Autodesk Fusion 360 part; units mm, degrees
note: some values were not read from the file. Set by a fixed rule: which sketch regions a step uses.
(part 2 of 2)
sketch "Sketch33" plane through (-2.5, 0, 0) normal (-1, 0, 0) x (0, 0, 1)
  circle A0 centre (22.5, 52.5) radius 3.5
  line L0 (35.5, 59.8175) -> (35.5, 45.1825)
  line L1 (35.5, 45.1825) -> (26.719, 52.5)
  line L2 (26.719, 52.5) -> (35.5, 59.8175)
  line L3 (9.5, 59.8175) -> (18.281, 52.5)
  line L4 (18.281, 52.5) -> (9.5, 45.1825)
  line L5 (9.5, 45.1825) -> (9.5, 59.8175)
  line L6 (29.8175, 39.5) -> (15.1825, 39.5)
  line L7 (15.1825, 39.5) -> (22.5, 48.281)
  line L8 (22.5, 48.281) -> (29.8175, 39.5)
  line L9 (22.5, 56.719) -> (15.1825, 65.5)
  line L10 (15.1825, 65.5) -> (29.8175, 65.5)
  line L11 (29.8175, 65.5) -> (22.5, 56.719)
  circle A1 centre (38.5, 65) radius 0.9
  circle A2 centre (6.5, 65) radius 0.9
  arc A3 (23.5, 4) -> (26, 1.5) centre (26, 4) ccw
  line L12 (23.5, 4) -> (23.5, 8.5)
  line L13 (23.5, 8.5) -> (6, 8.5)
  arc A4 (3.5, 11) -> (6, 8.5) centre (6, 11) ccw
  line L14 (3.5, 11) -> (3.5, 19)
  arc A5 (6, 21.5) -> (3.5, 19) centre (6, 19) ccw
  line L15 (6, 21.5) -> (26.5, 21.5)
  line L16 (26.5, 21.5) -> (26.5, 24)
  arc A6 (29, 26.5) -> (26.5, 24) centre (29, 24) ccw
  line L17 (29, 26.5) -> (39, 26.5)
  arc A7 (41.5, 24) -> (39, 26.5) centre (39, 24) ccw
  line L18 (41.5, 24) -> (41.5, 11)
  arc A8 (39, 8.5) -> (41.5, 11) centre (39, 11) ccw
  line L19 (39, 8.5) -> (36.5, 8.5)
  line L20 (36.5, 8.5) -> (36.5, 4)
  arc A9 (34, 1.5) -> (36.5, 4) centre (34, 4) ccw
  line L21 (34, 1.5) -> (46, 1.5)
  line L22 (46, 1.5) -> (46, 68.5)
  line L23 (46, 68.5) -> (-1.4, 68.5)
  line L24 (-1.4, 68.5) -> (-1.4, 1.5)
  line L25 (-1.4, 1.5) -> (26, 1.5)
  line L26 (24, 27) -> (11, 27)
  line L27 (11, 27) -> (11, 24)
  line L28 (11, 24) -> (24, 24)
  line L29 (24, 24) -> (24, 27)
  constraint horizontal L26
  constraint vertical L27
  constraint horizontal L28
  constraint vertical L29
extrude "Extrude39" cut sketch "Sketch33" against normal blind 5 contours L26 L27 L28 L29
sketch "Sketch34" plane through (0, 0, -2.9) normal (0, 0, -1) x (-1, 0, 0)
  line L0 (-37.85, 0) -> (-37.85, 1.5)
  line L1 (-37.85, 1.5) -> (-46.35, 1.5)
  line L2 (-46.35, 1.5) -> (-46.35, 68.5)
  line L3 (-46.35, 68.5) -> (1, 68.5)
  line L4 (1, 68.5) -> (1, 1.5)
  line L5 (1, 1.5) -> (-33.85, 1.5)
  line L6 (-33.85, 1.5) -> (-33.85, 0)
  line L7 (-33.85, 0) -> (2.85, 0)
  line L8 (2.85, 0) -> (2.85, 70)
  line L9 (2.85, 70) -> (-47.85, 70)
  line L10 (-47.85, 70) -> (-47.85, 0)
  line L11 (-47.85, 0) -> (-37.85, 0)
  line L12 (-46.35, 1.5) -> (-47.85, 1.5)
  constraint coincident L1.end L2.start
  constraint coincident L10 L12.end
  constraint perpendicular L10 L12
extrude "Extrude40" cut sketch "Sketch34" against normal blind 0.4 contours L0 L1 L10 L11 L12
sketch "Sketch35" plane through (0, 0, -2.9) normal (0, 0, -1) x (-1, 0, 0)
  line L0 (-47.85, 1.5) -> (-46.35, 1.5)
  line L1 (-46.35, 1.5) -> (-46.35, 68.5)
  line L2 (-46.35, 68.5) -> (1, 68.5)
  line L3 (1, 68.5) -> (1, 1.5)
  line L4 (1, 1.5) -> (-33.85, 1.5)
  line L5 (-33.85, 1.5) -> (-33.85, 0)
  line L6 (-33.85, 0) -> (2.85, 0)
  line L7 (2.85, 0) -> (2.85, 70)
  line L8 (2.85, 70) -> (-47.85, 70)
  line L9 (-47.85, 70) -> (-47.85, 1.5)
  line L10 (1, 1.5) -> (2.85, 1.5)
  constraint coincident L3.end L4.start
  constraint coincident L7 L10.end
  constraint perpendicular L7 L10
extrude "Extrude41" cut sketch "Sketch35" against normal blind 0.4 contours L4 L5 L6 L7 L10
sketch "Sketch36" plane through (0, 0, -2.9) normal (0, 0, -1) x (-1, 0, 0)
  line L0 (1, 1.5) -> (2.85, 1.5)
  line L1 (2.85, 1.5) -> (2.85, 70)
  line L2 (2.85, 70) -> (-47.85, 70)
  line L3 (-47.85, 70) -> (-47.85, 1.5)
  line L4 (-47.85, 1.5) -> (-46.35, 1.5)
  line L5 (-46.35, 1.5) -> (-46.35, 68.5)
  line L6 (-46.35, 68.5) -> (1, 68.5)
  line L7 (1, 68.5) -> (1, 1.5)
  line L8 (2.85, 2) -> (1, 2)
  dimension "d278" = 0.5
  constraint coincident L1 L8.start
  constraint coincident L7 L8.end
  constraint perpendicular L7 L8
  measures "d278" distance of L0 L8
extrude "Extrude42" cut sketch "Sketch36" against normal blind 0.4 contours L0 L1 L7 L8
sketch "Sketch37" plane through (0, 0, -2.9) normal (0, 0, -1) x (-1, 0, 0)
  line L0 (1, 2) -> (2.85, 2)
  line L1 (2.85, 2) -> (2.85, 70)
  line L2 (2.85, 70) -> (-47.85, 70)
  line L3 (-47.85, 70) -> (-47.85, 1.5)
  line L4 (-47.85, 1.5) -> (-46.35, 1.5)
  line L5 (-46.35, 1.5) -> (-46.35, 68.5)
  line L6 (-46.35, 68.5) -> (1, 68.5)
  line L7 (1, 68.5) -> (1, 2)
  line L8 (-46.35, 2) -> (-47.85, 2)
  dimension "d281" = 0.5
  constraint coincident L5 L8.start
  constraint coincident L3 L8.end
  constraint perpendicular L3 L8
  measures "d281" distance of L4 L8
extrude "Extrude43" cut sketch "Sketch37" against normal blind 0.4 contours L3 L4 L5 L8
sketch "Sketch38" plane through (0, 0, -2.5) normal (0, 0, -1) x (-1, 0, 0)
  circle A0 centre (-22.5, 17.5) radius 3.5
  circle A1 centre (-22.5, 52.5) radius 3.5
  line L0 (-18.281, 17.5) -> (-9.5, 24.8175)
  line L1 (-9.5, 24.8175) -> (-9.5, 10.1825)
  line L2 (-9.5, 10.1825) -> (-18.281, 17.5)
  line L3 (-15.1825, 39.5) -> (-29.8175, 39.5)
  line L4 (-29.8175, 39.5) -> (-22.5, 48.281)
  line L5 (-22.5, 48.281) -> (-15.1825, 39.5)
  line L6 (-29.8175, 65.5) -> (-15.1825, 65.5)
  line L7 (-15.1825, 65.5) -> (-22.5, 56.719)
  line L8 (-22.5, 56.719) -> (-29.8175, 65.5)
  line L9 (-22.5, 21.719) -> (-29.8175, 30.5)
  line L10 (-29.8175, 30.5) -> (-15.1825, 30.5)
  line L11 (-15.1825, 30.5) -> (-22.5, 21.719)
  line L12 (-15.1825, 4.5) -> (-29.8175, 4.5)
  line L13 (-29.8175, 4.5) -> (-22.5, 13.281)
  line L14 (-22.5, 13.281) -> (-15.1825, 4.5)
  line L15 (-18.281, 52.5) -> (-9.5, 59.8175)
  line L16 (-9.5, 59.8175) -> (-9.5, 45.1825)
  line L17 (-9.5, 45.1825) -> (-18.281, 52.5)
  line L18 (-35.5, 59.8175) -> (-26.719, 52.5)
  line L19 (-26.719, 52.5) -> (-35.5, 45.1825)
  line L20 (-35.5, 45.1825) -> (-35.5, 59.8175)
  line L21 (-35.5, 10.1825) -> (-35.5, 24.8175)
  line L22 (-35.5, 24.8175) -> (-26.719, 17.5)
  line L23 (-26.719, 17.5) -> (-35.5, 10.1825)
  line L24 (-37.85, 0) -> (-37.85, 2)
  line L25 (-37.85, 2) -> (-33.85, 2)
  line L26 (-33.85, 2) -> (-33.85, 0)
  line L27 (-33.85, 0) -> (2.85, 0)
  line L28 (2.85, 0) -> (2.85, 2)
  line L29 (2.85, 2) -> (1, 2)
  line L30 (1, 2) -> (1, 68.5)
  line L31 (1, 68.5) -> (-46.35, 68.5)
  line L32 (-46.35, 68.5) -> (-46.35, 2)
  line L33 (-46.35, 2) -> (-47.85, 2)
  line L34 (-47.85, 2) -> (-47.85, 0)
  line L35 (-47.85, 0) -> (-37.85, 0)
  line L36 (-47.85, 0) -> (-37.85, 0)
  line L37 (-37.85, 0) -> (-37.85, 2)
  line L38 (-37.85, 2) -> (-47.85, 2)
  line L39 (-47.85, 2) -> (-47.85, 0)
  line L40 (-33.85, 0) -> (2.85, 0)
  line L41 (2.85, 0) -> (2.85, 2)
  line L42 (2.85, 2) -> (-33.85, 2)
  line L43 (-33.85, 2) -> (-33.85, 0)
  dimension "d284" = 10
  dimension "d285" = 2
  dimension "d286" = 36.7
  constraint horizontal L36
  constraint vertical L37
  constraint horizontal L38
  constraint vertical L39
  constraint coincident L34.end L35.start
  constraint horizontal L40
  constraint vertical L41
  constraint horizontal L42
  constraint vertical L43
  constraint coincident L26.end L27.start
  measures "d284" distance of L34.end L24.start
  measures "d285" distance of L34.end L33.end
  measures "d286" distance of L26.end L27.end
extrude "Extrude44" add sketch "Sketch38" along normal blind 5 contours L24 L33 L34 L35 L36 L37 L38 L39 | L26 L27 L28 L29 L40 L41 L42 L43
sketch "Sketch39" plane through (0, 0, 47.85) normal (0, 0, 1) x (1, 0, 0)
  line L0 (46.35, 1.5) -> (-1.35, 1.5)
  line L1 (-1.35, 1.5) -> (-1.35, 68.5)
  line L2 (-1.35, 68.5) -> (46.35, 68.5)
  line L3 (46.35, 68.5) -> (46.35, 1.5)
  line L4 (-2.85, 70) -> (-2.85, 0)
  line L5 (-2.85, 0) -> (47.85, 0)
  line L6 (47.85, 0) -> (47.85, 70)
  line L7 (47.85, 70) -> (-2.85, 70)
  line L8 (-1.5, 2) -> (-2.85, 2)
  line L9 (-1.5, 2) -> (-1.35, 2)
  line L10 (46.35, 2) -> (47.85, 2)
  dimension "d289" = 2
  dimension "d290" = 2
  constraint coincident L4 L8.end
  constraint perpendicular L4 L8
  constraint coincident L1 L9.end
  constraint perpendicular L1 L9
  constraint coincident L3 L10.start
  constraint coincident L6 L10.end
  constraint perpendicular L6 L10
  measures "d289" distance of L5 L8
  measures "d290" distance of L5 L10
extrude "Extrude45" add sketch "Sketch39" along normal blind 5 contours L0 L1 L3 L4 L5 L6 L8 L9 L10
sketch "Sketch40" plane through (0, 2, 0) normal (0, 1, 0) x (-1, 0, 0)
  line L0 (2.85, -2.9) -> (1, -2.9)
  line L1 (1, -2.9) -> (1, -2.5)
  line L2 (1, -2.5) -> (-33.85, -2.5)
  line L3 (-33.85, -2.5) -> (-33.85, -7.5)
  line L4 (-33.85, -7.5) -> (2.85, -7.5)
  line L5 (2.85, -7.5) -> (2.85, -2.9)
  circle A0 centre (-30.95, -5) radius 1
  circle A1 centre (-14.05, -5) radius 1
  line L6 (-47.85, -2.9) -> (-47.85, -7.5)
  circle A2 centre (-14.05, 50.35) radius 1
  circle A3 centre (-30.95, 50.35) radius 1
  line L7 (-46.35, 52.85) -> (1.35, 52.85)
  line L8 (2.85, 47.85) -> (2.85, 52.85)
  line L9 (-47.85, 47.85) -> (-47.85, 52.85)
  dimension "d293" = 2
  dimension "d294" = 2
  dimension "d295" = 2.5
  dimension "d296" = 2.5
  dimension "d297" = 16.9
  dimension "d298" = 16.9
  dimension "d299" = 2
  dimension "d300" = 2
  dimension "d301" = 2.5
  dimension "d302" = 2.5
  dimension "d303" = 16.9
  dimension "d304" = 16.9
  measures "d293" diameter of A0
  measures "d294" diameter of A1
  measures "d295" distance of L4 A1.centre
  measures "d296" distance of L4 A0.centre
  measures "d297" distance of L5 A1.centre
  measures "d298" distance of A0.centre L6
  measures "d299" diameter of A2
  measures "d300" diameter of A3
  measures "d301" distance of A2.centre L7
  measures "d302" distance of A3.centre L7
  measures "d303" distance of A2.centre L8
  measures "d304" distance of A3.centre L9
extrude "Extrude46" cut sketch "Sketch40" against normal blind 5 contours A0 | A1 | A2 | A3
sketch "Sketch41" plane through (-2.5, 0, 0) normal (-1, 0, 0) x (0, 0, 1)
  line L0 (11, 27) -> (24, 27)
  line L1 (24, 27) -> (24, 24)
  line L2 (24, 24) -> (11, 24)
  line L3 (11, 24) -> (11, 27)
  circle A0 centre (22.5, 52.5) radius 3.5
  line L4 (35.5, 59.8175) -> (35.5, 45.1825)
  line L5 (35.5, 45.1825) -> (26.719, 52.5)
  line L6 (26.719, 52.5) -> (35.5, 59.8175)
  line L7 (9.5, 59.8175) -> (18.281, 52.5)
  line L8 (18.281, 52.5) -> (9.5, 45.1825)
  line L9 (9.5, 45.1825) -> (9.5, 59.8175)
  line L10 (29.8175, 39.5) -> (15.1825, 39.5)
  line L11 (15.1825, 39.5) -> (22.5, 48.281)
  line L12 (22.5, 48.281) -> (29.8175, 39.5)
  line L13 (22.5, 56.719) -> (15.1825, 65.5)
  line L14 (15.1825, 65.5) -> (29.8175, 65.5)
  line L15 (29.8175, 65.5) -> (22.5, 56.719)
  circle A1 centre (6.5, 65) radius 0.9
  circle A2 centre (38.5, 65) radius 0.9
  arc A3 (23.5, 4) -> (26, 1.5) centre (26, 4) ccw
  line L16 (23.5, 4) -> (23.5, 8.5)
  line L17 (23.5, 8.5) -> (6, 8.5)
  arc A4 (3.5, 11) -> (6, 8.5) centre (6, 11) ccw
  line L18 (3.5, 11) -> (3.5, 19)
  arc A5 (6, 21.5) -> (3.5, 19) centre (6, 19) ccw
  line L19 (6, 21.5) -> (26.5, 21.5)
  line L20 (26.5, 21.5) -> (26.5, 24)
  arc A6 (29, 26.5) -> (26.5, 24) centre (29, 24) ccw
  line L21 (29, 26.5) -> (39, 26.5)
  arc A7 (41.5, 24) -> (39, 26.5) centre (39, 24) ccw
  line L22 (41.5, 24) -> (41.5, 11)
  arc A8 (39, 8.5) -> (41.5, 11) centre (39, 11) ccw
  line L23 (39, 8.5) -> (36.5, 8.5)
  line L24 (36.5, 8.5) -> (36.5, 4)
  arc A9 (34, 1.5) -> (36.5, 4) centre (34, 4) ccw
  line L25 (34, 1.5) -> (46, 1.5)
  line L26 (46, 1.5) -> (46, 68.5)
  line L27 (46, 68.5) -> (-1.4, 68.5)
  line L28 (-1.4, 68.5) -> (-1.4, 1.5)
  line L29 (-1.4, 1.5) -> (26, 1.5)
  circle A10 centre (35, 40) radius 2
  dimension "d307" = 4
  measures "d307" diameter of A10
extrude "Extrude47" cut sketch "Sketch41" against normal blind 3 contours A10
sketch "Sketch42" plane through (-2.5, 0, 0) normal (-1, 0, 0) x (0, 0, 1)
  circle A0 centre (35, 40) radius 2
  line L0 (11, 27) -> (24, 27)
  line L1 (24, 27) -> (24, 24)
  line L2 (24, 24) -> (11, 24)
  line L3 (11, 24) -> (11, 27)
  circle A1 centre (22.5, 52.5) radius 3.5
  line L4 (35.5, 59.8175) -> (35.5, 45.1825)
  line L5 (35.5, 45.1825) -> (26.719, 52.5)
  line L6 (26.719, 52.5) -> (35.5, 59.8175)
  line L7 (9.5, 59.8175) -> (18.281, 52.5)
  line L8 (18.281, 52.5) -> (9.5, 45.1825)
  line L9 (9.5, 45.1825) -> (9.5, 59.8175)
  line L10 (29.8175, 39.5) -> (15.1825, 39.5)
  line L11 (15.1825, 39.5) -> (22.5, 48.281)
  line L12 (22.5, 48.281) -> (29.8175, 39.5)
  line L13 (22.5, 56.719) -> (15.1825, 65.5)
  line L14 (15.1825, 65.5) -> (29.8175, 65.5)
  line L15 (29.8175, 65.5) -> (22.5, 56.719)
  circle A2 centre (6.5, 65) radius 0.9
  circle A3 centre (38.5, 65) radius 0.9
  arc A4 (23.5, 4) -> (26, 1.5) centre (26, 4) ccw
  line L16 (23.5, 4) -> (23.5, 8.5)
  line L17 (23.5, 8.5) -> (6, 8.5)
  arc A5 (3.5, 11) -> (6, 8.5) centre (6, 11) ccw
  line L18 (3.5, 11) -> (3.5, 19)
  arc A6 (6, 21.5) -> (3.5, 19) centre (6, 19) ccw
  line L19 (6, 21.5) -> (26.5, 21.5)
  line L20 (26.5, 21.5) -> (26.5, 24)
  arc A7 (29, 26.5) -> (26.5, 24) centre (29, 24) ccw
  line L21 (29, 26.5) -> (39, 26.5)
  arc A8 (41.5, 24) -> (39, 26.5) centre (39, 24) ccw
  line L22 (41.5, 24) -> (41.5, 11)
  arc A9 (39, 8.5) -> (41.5, 11) centre (39, 11) ccw
  line L23 (39, 8.5) -> (36.5, 8.5)
  line L24 (36.5, 8.5) -> (36.5, 4)
  arc A10 (34, 1.5) -> (36.5, 4) centre (34, 4) ccw
  line L25 (34, 1.5) -> (46, 1.5)
  line L26 (46, 1.5) -> (46, 68.5)
  line L27 (46, 68.5) -> (-1.4, 68.5)
  line L28 (-1.4, 68.5) -> (-1.4, 1.5)
  line L29 (-1.4, 1.5) -> (26, 1.5)
  line L30 (46, 68.5) -> (37, 68.5)
  line L31 (37, 68.5) -> (37, 61)
  line L32 (37, 61) -> (46, 61)
  line L33 (46, 61) -> (46, 68.5)
  constraint horizontal L30
  constraint vertical L31
  constraint horizontal L32
  constraint vertical L33
  constraint coincident L26.end L27.start
extrude "Extrude48" add sketch "Sketch42" along normal blind 9 contours A3 | L26 L27 L30 L31 L32 L33
sketch "Sketch43" plane through (0, 68.5, 0) normal (0, 1, 0) x (-1, 0, 0)
  line L0 (2.85, 46) -> (2.85, 37)
  line L1 (2.85, 37) -> (11.5, 37)
  line L2 (11.5, 37) -> (11.5, 46)
  line L3 (11.5, 46) -> (2.85, 46)
  circle A0 centre (7, 41.5) radius 2.675
  dimension "d312" = 5.35
  dimension "d313" = 4.5
  dimension "d314" = 4.5
  measures "d312" diameter of A0
  measures "d313" distance of L1 A0.centre
  measures "d314" distance of L2 A0.centre
extrude "Extrude49" cut sketch "Sketch43" against normal blind 9 contours A0
fillet "Fillet15" radius 2 1 edges at (-11.5, 64.75, 46)
fillet "Fillet16" radius 2 1 edges at (-11.5, 64.75, 37)
fillet "Fillet17" radius 2 1 edges at (-2.5, 64.75, 37)
fillet "Fillet18" radius 1 1 edges at (-2.85, 64.75, 46)
equation "d297 = ( 50.7 / 3 ) * 1 mm"
equation "d298 = ( 50.7 / 3 ) * 1 mm"
equation "d303 = ( 50.7 / 3 ) * 1 mm"
equation "d304 = ( 50.7 / 3 ) * 1 mm"
